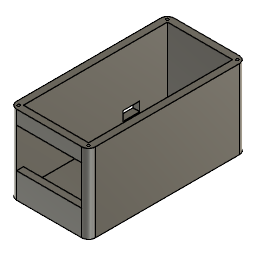
box (Autodesk Fusion 360 design; units mm, degrees)
Autodesk Fusion 360 part; units mm, degrees
sketch "Sketch1" plane through (0, 0, 0) normal (0, 0, 1) x (1, 0, 0)
  line L0 (-50.8, 101.6) -> (50.8, 101.6)
  line L1 (50.8, 101.6) -> (50.8, -101.6)
  line L2 (50.8, -101.6) -> (-50.8, -101.6)
  line L3 (-50.8, -101.6) -> (-50.8, 101.6)
  line L4 (0, 0) -> (0, 101.6) construction
  line L5 (0, 0) -> (50.8, 0) construction
  dimension "d1" = 101.6
  dimension "d2" = 203.2
  constraint horizontal L0
  constraint vertical L1
  constraint horizontal L2
  constraint vertical L3
  constraint coincident L4.start L5.start
  constraint midpoint L0 L4.end
  constraint vertical L4
  constraint midpoint L1 L5.end
  constraint horizontal L5
  measures "d1" distance of L0.start L0.end
  measures "d2" distance of L0.start L2.end
extrude "Extrude1" add sketch "Sketch1" along normal blind 101.6
shell "Shell1" thickness 8.89 removed faces 1 at (-16.9333, -33.8667, 101.6)
sketch "Sketch3" plane through (0, -101.6, 0) normal (0, -1, 0) x (1, 0, 0)
  line L0 (-50.8, 0) -> (50.8, 0)
  line L1 (50.8, 0) -> (50.8, 101.6)
  line L2 (50.8, 101.6) -> (-50.8, 101.6)
  line L3 (-50.8, 101.6) -> (-50.8, 0)
  line L4 (-41.91, 83.82) -> (41.91, 83.82)
  line L5 (41.91, 83.82) -> (41.91, 33.02)
  line L6 (41.91, 33.02) -> (-41.91, 33.02)
  line L7 (-41.91, 33.02) -> (-41.91, 83.82)
  line L8 (0, 101.6) -> (0, 83.82) construction
  line L9 (41.91, 8.89) -> (-41.91, 8.89)
  line L10 (-41.91, 8.89) -> (-41.91, 101.6)
  line L11 (-41.91, 101.6) -> (41.91, 101.6)
  line L12 (41.91, 101.6) -> (41.91, 8.89)
  point P0 (0, 83.82)
  point P1 (0, 58.42)
  point P2 (-41.91, 58.42)
  point P3 (41.91, 58.42)
  dimension "d15" = 50.8
  dimension "d20" = 25.4
  dimension "d21" = 58.42
  dimension "d25" = 25.4
  constraint horizontal L4
  constraint vertical L5
  constraint horizontal L6
  constraint vertical L7
  constraint coincident L4 P0
  constraint midpoint L4 P0
  constraint midpoint L2 L8.start
  constraint coincident P0 L8.end
  constraint vertical L8
  constraint midpoint L7 P2
  constraint midpoint L5 P3
  constraint coincident L12 P3
  measures "d15" distance of L4.start L6.end
  measures "d20" distance of P0 P1
  measures "d21" distance of L0 P1
  measures "d25" distance of L6 P1
extrude "Extrude3" cut sketch "Sketch3" against normal blind 12.7 contours L4 L5 L6 L7 L10 L12
fillet "Fillet1" radius 8.89 4 edges at (-50.8, -101.6, 50.8) (50.8, -101.6, 50.8) (-50.8, 101.6, 50.8) (50.8, 101.6, 50.8)
sketch "Sketch4" plane through (0, 0, 101.6) normal (0, 0, 1) x (-1, 0, 0)
  arc A0 (-50.8, -92.71) -> (-41.91, -101.6) centre (-41.91, -92.71) ccw
  line L0 (-41.91, -101.6) -> (41.91, -101.6)
  arc A1 (41.91, -101.6) -> (50.8, -92.71) centre (41.91, -92.71) ccw
  line L1 (50.8, -92.71) -> (50.8, 92.71)
  arc A2 (50.8, 92.71) -> (41.91, 101.6) centre (41.91, 92.71) ccw
  line L2 (41.91, 101.6) -> (-41.91, 101.6)
  arc A3 (-41.91, 101.6) -> (-50.8, 92.71) centre (-41.91, 92.71) ccw
  line L3 (-50.8, 92.71) -> (-50.8, -92.71)
  line L4 (41.91, 92.71) -> (41.91, -92.71)
  line L5 (41.91, -92.71) -> (-41.91, -92.71)
  line L6 (-41.91, -92.71) -> (-41.91, 92.71)
  line L7 (-41.91, 92.71) -> (41.91, 92.71)
  line L8 (41.91, 92.71) -> (48.1962, 98.9962) construction
  arc A4 (41.91, 101.6) -> (50.8, 92.71) centre (53.2921, 104.0921) ccw construction
  circle A5 centre (45.0531, 95.8531) radius 1.778
  line L9 (41.91, 92.71) -> (41.91, -92.71)
  line L10 (41.91, -92.71) -> (41.91, 92.71)
  line L11 (41.91, 92.71) -> (41.91, 101.6)
  line L12 (41.91, 101.6) -> (41.91, 92.71)
  line L13 (-41.91, 92.71) -> (-48.1962, 98.9962) construction
  arc A6 (-50.8, 92.71) -> (-41.91, 101.6) centre (-53.2921, 104.0921) ccw construction
  circle A7 centre (-45.0531, 95.8531) radius 1.778
  line L14 (50.8, 0) -> (-50.8, 0) construction
  point P0 (45.0531, 95.8531)
  point P1 (46.3103, 97.1103)
  point P2 (43.7959, 94.5959)
  point P3 (-43.7959, 94.5959)
  point P4 (-46.3103, 97.1103)
  dimension "d26" = 3.556
  dimension "d29" = 3.556
  constraint coincident A2.centre L4.start
  constraint midpoint A2 L8.end
  constraint midpoint L8 P0
  constraint coincident P0 A4
  constraint coincident A2.end L2.start
  constraint coincident L1.end A2.start
  constraint coincident P0 A5.centre
  constraint coincident A3.centre L6.end
  constraint midpoint A3 L13.end
  constraint coincident L2.end A3.start
  constraint coincident A3.end L3.start
  constraint midpoint A6 A7.centre
  constraint horizontal P0 A7.centre
  constraint midpoint L1 L14.start
  constraint midpoint L3 L14.end
  constraint coincident L8 P1
  constraint coincident A5 P1
  constraint coincident A5 P2
  constraint coincident L8 P2
  constraint coincident A7 P3
  constraint coincident L13 P3
  constraint coincident L13 P4
  constraint coincident A7 P4
  measures "d26" diameter of A5
  measures "d29" diameter of A7
extrude "Extrude4" cut sketch "Sketch4" against normal blind 14.732 contours A5 | A7
mirror "Mirror1" about plane through (0, 0, 0) normal (0, 1, 0) of "Extrude4"
sketch "Sketch5" plane through (0, 0, 8.89) normal (0, 0, 1) x (-1, 0, 0)
  line L0 (41.91, 92.71) -> (-41.91, 92.71)
  line L1 (-41.91, 92.71) -> (-41.91, -92.71)
  line L2 (-41.91, -92.71) -> (41.91, -92.71)
  line L3 (41.91, -92.71) -> (41.91, 92.71)
  line L4 (-26.67, -57.785) -> (-26.67, 57.785)
  line L5 (-26.67, -57.785) -> (-41.91, -57.785)
  line L6 (-26.67, 57.785) -> (-41.91, 57.785)
  line L7 (-41.91, 57.785) -> (-41.91, 62.865)
  line L8 (-21.59, -57.785) -> (-21.59, 57.785)
  line L9 (-21.59, 57.785) -> (-21.59, 62.865)
  line L10 (-21.59, 62.865) -> (-41.91, 62.865)
  line L11 (-21.59, -57.785) -> (-21.59, -62.865)
  line L12 (-21.59, -62.865) -> (-41.91, -62.865)
  line L13 (-41.91, -62.865) -> (-41.91, -57.785)
  line L14 (41.91, 0) -> (-21.59, 0) construction
  line L15 (-21.59, 62.865) -> (-21.59, 92.71) construction
  point P0 (-26.67, 0)
  point P1 (-21.59, 0)
  dimension "d33" = 115.57
  dimension "d34" = 15.24
  dimension "d36" = 5.08
  dimension "d37" = 115.57
  dimension "d38" = 5.08
  dimension "d39" = 5.08
  dimension "d40" = 5.08
  dimension "d41" = 63.5
  dimension "d44" = 29.845
  constraint parallel L1 L4
  constraint midpoint L4 P0
  constraint coincident L1 L5.end
  constraint perpendicular L1 L5
  constraint coincident L1 L6.end
  constraint perpendicular L1 L6
  constraint vertical L7
  constraint vertical L8
  constraint midpoint L8 P1
  constraint horizontal P0 P1
  constraint parallel L8 L9
  constraint parallel L8 L11
  constraint coincident L1 L12.end
  constraint perpendicular L1 L12
  constraint midpoint L3 L14.start
  constraint coincident P1 L14.end
  constraint perpendicular L8 L14
  constraint coincident L0 L15.end
  constraint perpendicular L0 L15
  measures "d33" distance of L4.start L4.end
  measures "d34" distance of L1 L4
  measures "d36" distance of L6.end L7.end
  measures "d37" distance of L8.start L8.end
  measures "d38" distance of L4 L8
  measures "d39" distance of L8.end L9.end
  measures "d40" distance of L8.start L11.end
  measures "d41" distance of L14.start P1
  measures "d44" distance of L9.end L15.end
extrude "Extrude5" add sketch "Sketch5" along normal blind 50.8 contours L1 L4 L5 L6 L7 L8 L9 L10 L11 L12 L13
sketch "Sketch6" plane through (0, 62.865, 0) normal (0, 1, 0) x (-1, 0, 0)
  line L0 (-41.91, 8.89) -> (-21.59, 8.89)
  line L1 (-21.59, 8.89) -> (-21.59, 59.69)
  line L2 (-21.59, 59.69) -> (-41.91, 59.69)
  line L3 (-41.91, 59.69) -> (-41.91, 8.89)
  line L4 (-38.1, 36.9147) -> (-30.48, 36.9147)
  line L5 (-30.48, 36.9147) -> (-30.48, 24.2147)
  line L6 (-30.48, 24.2147) -> (-38.1, 24.2147)
  line L7 (-38.1, 24.2147) -> (-38.1, 36.9147)
  line L8 (-38.1, 36.9147) -> (-30.48, 24.2147) construction
  line L9 (-38.1, 24.2147) -> (-30.48, 36.9147) construction
  line L10 (-21.59, 59.69) -> (-41.91, 59.69)
  line L11 (-41.91, 59.69) -> (-26.67, 59.69)
  line L12 (-26.67, 59.69) -> (-41.91, 59.69)
  line L13 (-41.91, 59.69) -> (-21.59, 59.69)
  line L14 (-26.67, 59.69) -> (-26.67, 8.89) construction
  line L15 (-41.91, 30.5647) -> (-26.67, 30.5647) construction
  line L16 (-41.91, 59.69) -> (-26.67, 59.69) construction
  line L17 (-34.29, 59.69) -> (-34.29, 8.89) construction
  point P0 (-34.29, 30.5647)
  dimension "d45" = 7.62
  dimension "d46" = 12.7
  dimension "d51" = 15.3247
  constraint horizontal L4
  constraint vertical L5
  constraint horizontal L6
  constraint vertical L7
  constraint midpoint P0 L8
  constraint coincident L11.end L12.start
  constraint coincident L0 L14.end
  constraint vertical L14
  constraint coincident L3 L15.start
  constraint coincident L14 L15.end
  constraint horizontal L15
  constraint midpoint P0 L15
  constraint coincident L2.end L3.start
  constraint midpoint L16 L17.start
  constraint coincident L0 L17.end
  constraint vertical L17
  measures "d45" distance of L4.start L4.end
  measures "d46" distance of L4.start L6.end
  measures "d51" distance of L0 L6
extrude "Extrude6" cut sketch "Sketch6" against normal blind 5.08 contours L4 L5 L6 L7
sketch "Sketch7" plane through (-50.8, 0, 0) normal (-1, 0, 0) x (0, -1, 0)
  line L0 (-92.71, 101.6) -> (-92.71, 0)
  line L1 (-92.71, 0) -> (92.71, 0)
  line L2 (92.71, 0) -> (92.71, 101.6)
  line L3 (92.71, 101.6) -> (-92.71, 101.6)
  line L4 (-57.105, 31.4) -> (-35.605, 31.4)
  line L5 (-35.605, 31.4) -> (-35.605, 19.4)
  line L6 (-35.605, 19.4) -> (-57.105, 19.4)
  line L7 (-57.105, 19.4) -> (-57.105, 31.4)
  line L8 (-92.71, 50.8) -> (0, 50.8) construction
  line L9 (0, 50.8) -> (0, 0) construction
  line L10 (-57.105, 31.4) -> (-35.605, 19.4) construction
  line L11 (-35.605, 31.4) -> (-57.105, 19.4) construction
  line L12 (-46.355, 50.8) -> (-46.355, 0) construction
  line L13 (0, 25.4) -> (-92.71, 25.4) construction
  point P0 (-46.355, 25.4)
  point P1 (-46.355, 25.4)
  dimension "d52" = 21.5
  dimension "d53" = 12
  constraint horizontal L4
  constraint vertical L5
  constraint horizontal L6
  constraint vertical L7
  constraint midpoint L0 L8.start
  constraint perpendicular L0 L8
  constraint coincident L9.end origin
  constraint perpendicular L1 L9
  constraint midpoint L10 P1
  constraint midpoint L8 L12.start
  constraint coincident L1 L12.end
  constraint perpendicular L1 L12
  constraint midpoint L9 L13.start
  constraint coincident L0 L13.end
  constraint perpendicular L0 L13
  constraint midpoint L13 P1
  constraint coincident P1 P0
  measures "d52" distance of L4.start L4.end
  measures "d53" distance of L4.start L6.end
extrude "Extrude7" cut sketch "Sketch7" against normal blind 10 contours L4 L5 L6 L7
